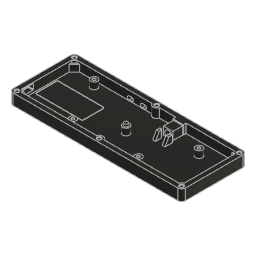
HTangl V2 Case (Autodesk Fusion 360 design; units mm, degrees)
Autodesk Fusion 360 part; units mm, degrees
sketch "Main Case" plane through (0, 0, 0) normal (0, 0, 1) x (1, 0, 0)
  line L0 (411.2, 144.2) -> (411.2, 21.8)
  line L1 (52.8, 13.8) -> (403.2, 13.8)
  line L2 (44.8, 21.8) -> (44.8, 144.2)
  circle A0 centre (228, 144.2) radius 3.3
  line L3 (237, 135.2) -> (219, 135.2)
  line L4 (237, 135.2) -> (237, 141)
  line L5 (219, 135.2) -> (219, 141)
  line L6 (403.2, 152.2) -> (52.8, 152.2)
  circle A1 centre (403.2, 144.2) radius 3.3
  line L7 (235.6916, 142) -> (395.5084, 142)
  arc A2 (395.5084, 142) -> (401, 136.5084) centre (403.2, 144.2) ccw
  arc A3 (411.2, 144.2) -> (403.2, 152.2) centre (403.2, 144.2) ccw
  arc A4 (220.3084, 142) -> (235.6916, 142) centre (228, 144.2) ccw
  circle A5 centre (52.8, 144.2) radius 3.3
  line L8 (220.3084, 142) -> (60.4916, 142)
  arc A6 (52.8, 152.2) -> (44.8, 144.2) centre (52.8, 144.2) ccw
  arc A7 (55, 136.5084) -> (60.4916, 142) centre (52.8, 144.2) ccw
  circle A8 centre (52.8, 21.8) radius 3.3
  line L9 (55, 136.5084) -> (55, 29.4916)
  arc A9 (44.8, 21.8) -> (52.8, 13.8) centre (52.8, 21.8) ccw
  arc A10 (60.4916, 24) -> (55, 29.4916) centre (52.8, 21.8) ccw
  circle A11 centre (403.2, 21.8) radius 3.3
  line L10 (401, 136.5084) -> (401, 29.4916)
  arc A12 (401, 29.4916) -> (395.5084, 24) centre (403.2, 21.8) ccw
  arc A13 (403.2, 13.8) -> (411.2, 21.8) centre (403.2, 21.8) ccw
  circle A14 centre (228, 21.8) radius 3.3
  line L11 (60.4916, 24) -> (220.3084, 24)
  line L12 (395.5084, 24) -> (235.6916, 24)
  arc A15 (235.6916, 24) -> (220.3084, 24) centre (228, 21.8) ccw
  line L13 (237, 30.8) -> (219, 30.8)
  line L14 (237, 30.8) -> (237, 25)
  line L15 (219, 30.8) -> (219, 25)
  line L16 (237, 141) -> (393, 141)
  line L17 (393, 141) -> (400, 134)
  line L18 (237, 25) -> (393, 25)
  line L19 (393, 25) -> (400, 32)
  line L20 (400, 32) -> (400, 134)
  line L21 (219, 25) -> (63, 25)
  line L22 (219, 141) -> (63, 141)
  line L23 (63, 141) -> (56, 134)
  line L24 (56, 134) -> (56, 32)
  line L25 (56, 32) -> (63, 25)
  point P0 (403.2, 144.2)
  point P1 (52.8, 144.2)
  point P2 (52.8, 21.8)
  point P3 (403.2, 21.8)
  dimension "d151" = 6.6
  dimension "d158" = 6.6
  dimension "d162" = 8
  dimension "d168" = 6.6
  dimension "d169" = 16
  dimension "d172" = 6.6
  dimension "d173" = 16
  dimension "d176" = 6.6
  dimension "d177" = 16
  dimension "d179" = 6.6
  dimension "d180" = 16
  dimension "d183" = 18
  dimension "d187" = 156
  dimension "d188" = 156
  dimension "d189" = 156
  dimension "d190" = 156
  dimension "d191" = 102
  constraint vertical L0
  constraint perpendicular L0 L1
  constraint perpendicular L1 L2
  constraint perpendicular L3 L4
  constraint perpendicular L3 L5
  constraint perpendicular L2 L6
  constraint coincident P0 A1.centre
  constraint horizontal L7
  constraint tangent L6 A3
  constraint tangent L0 A3
  constraint concentric A0 A4
  constraint coincident P1 A5.centre
  constraint concentric A5 A6
  constraint parallel L6 L8
  constraint coincident A7.start A6
  constraint concentric A6 A7
  constraint coincident P2 A8.centre
  constraint concentric A8 A9
  constraint coincident A10.start A9
  constraint concentric A9 A10
  constraint coincident P3 A11.centre
  constraint perpendicular L7 L10
  constraint concentric A12 A13
  constraint concentric A14 A15
  constraint horizontal L11
  constraint parallel L11 L12
  constraint perpendicular L13 L15
  constraint perpendicular L4 L16
  constraint perpendicular L14 L18
  constraint perpendicular L18 L20
  constraint perpendicular L15 L21
  constraint perpendicular L5 L22
  constraint perpendicular L22 L24
  measures "d151" diameter of A0
  measures "d158" diameter of A1
  measures "d162" radius of A3
  measures "d168" diameter of A5
  measures "d169" diameter of A6
  measures "d172" diameter of A8
  measures "d173" diameter of A9
  measures "d176" diameter of A11
  measures "d177" diameter of A12
  measures "d179" diameter of A14
  measures "d180" diameter of A15
  measures "d183" distance of L13.start L13.end
  measures "d187" distance of L4.end L16.end
  measures "d188" distance of L14.end L18.end
  measures "d189" distance of L15.end L21.end
  measures "d190" distance of L5.end L22.end
  measures "d191" distance of L23.end L24.end
extrude "Case Bottom" add sketch "Main Case" along normal blind 4.2 contours L3 L4 L5 L13 L14 L15 L16 L17 L18 L19 L20 L21 L22 L23 L24 L25 | L7 A2 A4 L8 A7 L9 A10 L10 A12 L11 L12 A15 makes body 1
sketch "Standoffs" plane through (0, 0, 4.2) normal (0, 0, 1) x (-1, 0, 0)
  circle A0 centre (-228, -79) radius 7.2
  circle A1 centre (-109, -130) radius 7.3
  circle A2 centre (-159, -35) radius 7.3
  circle A3 centre (-298, -35) radius 7.3
  circle A4 centre (-347, -115) radius 7.3
  circle A5 centre (-228, -79) radius 4.05
  circle A6 centre (-109, -130) radius 2.6
  circle A7 centre (-159, -35) radius 2.6
  circle A8 centre (-298, -35) radius 2.6
  circle A9 centre (-347, -115) radius 2.6
  point P0 (-228, -79)
  point P1 (-347, -115)
  point P2 (-298, -35)
  point P3 (-159, -35)
  point P4 (-109, -130)
  dimension "d35" = 14.4
  dimension "d36" = 14.6
  dimension "d37" = 14.6
  dimension "d38" = 14.6
  dimension "d39" = 14.6
  dimension "d41" = 8.1
  dimension "d62" = 5.2
  dimension "d63" = 5.2
  dimension "d64" = 5.2
  dimension "d65" = 5.2
  constraint coincident P0 A0.centre
  constraint coincident P4 A1.centre
  constraint coincident P3 A2.centre
  constraint coincident P2 A3.centre
  constraint coincident P1 A4.centre
  constraint concentric A2 A7
  constraint concentric A4 A9
  measures "d35" diameter of A0
  measures "d36" diameter of A1
  measures "d37" diameter of A2
  measures "d38" diameter of A3
  measures "d39" diameter of A4
  measures "d41" diameter of A5
  measures "d62" diameter of A6
  measures "d63" diameter of A7
  measures "d64" diameter of A8
  measures "d65" diameter of A9
extrude "Case Standoffs" add sketch "Standoffs" along normal blind 14.1 bodies 1
extrude "Center Post" add sketch "Standoffs" along normal blind 19.2 contours A5 bodies 1
extrude "Case Walls" add sketch "Main Case" along normal blind 23.4 contours L0 L1 L2 L6 A3 A6 A9 A13 bodies 1
extrude "PCB Mounting Holes" add 4 faces at (346.3647, 114.1522, 4.2) (297.2192, 35.376, 4.2) (159.7161, 35.7466, 4.2) (109.2885, 130.6201, 4.2) along direction (0, 0, 1) blind 10.2 on bodies 1 bodies 1
fillet "PCB Mounting Hole Fillet" radius 0.6 4 edges at (349.4241, 114.0598, 18.3) (300.4241, 34.0598, 18.3) (161.4241, 34.0598, 18.3) (111.4241, 129.0598, 18.3) on bodies 1
extrude "Top Panel Mounting Holes 1" add sketch "Main Case" along normal blind 12.6 contours A0 | A1 | A5 | A8 | A11 | A14 bodies 1
sketch "Top Panel Bolt Inset" plane through (0, 0, 23.4) normal (0, 0, 1) x (-1, 0, 0)
  line L0 (-60.4916, -142) -> (-220.3084, -142)
  arc A0 (-220.3084, -142) -> (-235.6916, -142) centre (-228, -144.2) ccw
  line L1 (-235.6916, -142) -> (-395.5084, -142)
  arc A1 (-395.5084, -142) -> (-401, -136.5084) centre (-403.2, -144.2) ccw
  line L2 (-401, -136.5084) -> (-401, -29.4916)
  arc A2 (-401, -29.4916) -> (-395.5084, -24) centre (-403.2, -21.8) ccw
  line L3 (-395.5084, -24) -> (-235.6916, -24)
  arc A3 (-235.6916, -24) -> (-220.3084, -24) centre (-228, -21.8) ccw
  line L4 (-220.3084, -24) -> (-60.4916, -24)
  arc A4 (-60.4916, -24) -> (-55, -29.4916) centre (-52.8, -21.8) ccw
  line L5 (-55, -29.4916) -> (-55, -136.5084)
  arc A5 (-55, -136.5084) -> (-60.4916, -142) centre (-52.8, -144.2) ccw
  circle A6 centre (-52.8, -144.2) radius 3.3
  circle A7 centre (-228, -144.2) radius 3.3
  circle A8 centre (-228, -21.8) radius 3.3
  circle A9 centre (-403.2, -144.2) radius 3.3
  circle A10 centre (-52.8, -21.8) radius 3.3
  circle A11 centre (-403.2, -21.8) radius 3.3
  arc A12 (-44.8, -21.8) -> (-52.8, -13.8) centre (-52.8, -21.8) ccw
  line L6 (-52.8, -13.8) -> (-403.2, -13.8)
  arc A13 (-403.2, -13.8) -> (-411.2, -21.8) centre (-403.2, -21.8) ccw
  line L7 (-411.2, -21.8) -> (-411.2, -144.2)
  arc A14 (-411.2, -144.2) -> (-403.2, -152.2) centre (-403.2, -144.2) ccw
  line L8 (-403.2, -152.2) -> (-52.8, -152.2)
  arc A15 (-52.8, -152.2) -> (-44.8, -144.2) centre (-52.8, -144.2) ccw
  line L9 (-44.8, -144.2) -> (-44.8, -21.8)
  circle A16 centre (-52.8, -144.2) radius 4.5
  circle A17 centre (-228, -144.2) radius 4.5
  circle A18 centre (-403.2, -144.2) radius 4.5
  circle A19 centre (-403.2, -21.8) radius 4.5
  circle A20 centre (-228, -21.8) radius 4.5
  circle A21 centre (-52.8, -21.8) radius 4.5
  dimension "d196" = 9
  dimension "d197" = 9
  dimension "d198" = 9
  dimension "d199" = 9
  dimension "d200" = 9
  dimension "d201" = 9
  constraint concentric A5 A16
  constraint concentric A0 A17
  constraint concentric A1 A18
  constraint concentric A2 A19
  constraint concentric A3 A20
  constraint concentric A4 A21
  measures "d196" diameter of A16
  measures "d197" diameter of A17
  measures "d198" diameter of A18
  measures "d199" diameter of A19
  measures "d200" diameter of A20
  measures "d201" diameter of A21
extrude "Top Panel Bolt Inset (1)" cut sketch "Top Panel Bolt Inset" against normal blind 1.2 contours A16 | A17 | A18 | A19 | A20 | A21 bodies 1
sketch "GC Port" plane through (0, 142, 0) normal (0, -1, 0) x (1, 0, 0)
  line L0 (235.6916, 4.2) -> (395.5084, 4.2)
  line L1 (395.5084, 4.2) -> (395.5084, 23.4)
  line L2 (235.6916, 23.4) -> (235.6916, 4.2)
  line L3 (271.55, 21.1) -> (291.45, 21.1)
  line L4 (271.55, 21.1) -> (271.55, 4.2)
  line L5 (291.45, 21.1) -> (291.45, 4.2)
  line L6 (291.45, 4.2) -> (291.45, 3.2)
  line L7 (271.55, 4.2) -> (271.55, 3.2)
  line L8 (291.45, 4.2) -> (271.55, 4.2)
  circle A0 centre (281.5, 11.25) radius 7.25
  line L9 (291.45, 3.2) -> (271.55, 3.2)
  line L10 (276.6624, 5.85) -> (286.3376, 5.85)
  point P0 (281.5, 6.05)
  point P1 (281.5, 5.85)
  dimension "d290" = 1
  dimension "d394" = 14.5
  dimension "d396" = 0.2
  constraint horizontal L3
  constraint coincident L0 L4.end
  constraint perpendicular L0 L4
  constraint coincident L0 L5.end
  constraint perpendicular L0 L5
  constraint perpendicular L7 L9
  constraint coincident A0 L10.start
  constraint coincident A0 L10.end
  constraint horizontal L10
  measures "d290" distance of L5.end L6.end
  measures "d394" diameter of A0
  measures "d396" distance of P0 P1
extrude "GC Port Cutout" cut sketch "GC Port" against normal blind 10.2 bodies 1
extrude "GC Port Surround" add sketch "GC Port" along normal blind 27 separate body contours L0 L3 L4 L5 L8 A0 | L0 L6 L7 L8 A0 L9 | L0 L8 A0 L10 | L0 L8 A0 makes body 2
extrude "GC Port Inset" cut sketch "GC Port" along normal blind 2.1 bodies 1 2
sketch "GC Port 2" plane through (0, 142, 0) normal (0, -1, 0) x (1, 0, 0)
  line L0 (271.55, 4.2) -> (271.55, 21.1)
  line L1 (271.55, 21.1) -> (291.45, 21.1)
  line L2 (291.45, 21.1) -> (291.45, 4.2)
  line L3 (291.45, 4.2) -> (395.5084, 4.2)
  line L4 (395.5084, 4.2) -> (395.5084, 23.4)
  line L5 (395.5084, 23.4) -> (235.6916, 23.4)
  line L6 (235.6916, 23.4) -> (235.6916, 4.2)
  line L7 (271.55, 21.1) -> (271.55, 4.2)
  line L8 (271.55, 21.1) -> (291.45, 21.1)
  line L9 (291.45, 21.1) -> (291.45, 4.2)
  line L10 (291.45, 4.2) -> (292.65, 4.2)
  line L11 (271.55, 4.2) -> (270.35, 4.2)
  line L12 (270.35, 4.2) -> (270.35, 23.4)
  line L13 (270.35, 23.4) -> (292.65, 23.4)
  line L14 (292.65, 23.4) -> (292.65, 4.2)
  line L15 (235.6916, 4.2) -> (271.55, 4.2)
  dimension "d322" = 1.2
  dimension "d323" = 1.2
  dimension "d324" = 22.3
  constraint coincident L0.end L1.start
  constraint coincident L1.end L2.start
  constraint coincident L0.start L7.end
  constraint coincident L2.end L3.start
  constraint perpendicular L9 L10
  constraint perpendicular L7 L11
  constraint coincident L5 L12.end
  constraint perpendicular L5 L12
  constraint perpendicular L12 L13
  measures "d322" distance of L2.end L10.end
  measures "d323" distance of L0.start L11.end
  measures "d324" distance of L12.end L13.end
extrude "GC Port Surround 2" add sketch "GC Port 2" along normal blind 6 contours L0 L1 L2 L3 L5 L7 L8 L9 L10 L11 L12 L13 L14 L15 bodies 1 2
sketch "GC Port 3" plane through (0, 152.2, 0) normal (0, 1, 0) x (-1, 0, 0)
  line L0 (-291.45, 3.2) -> (-291.45, 21.1)
  line L1 (-291.45, 21.1) -> (-271.55, 21.1)
  line L2 (-271.55, 21.1) -> (-271.55, 3.2)
  line L3 (-403.2, 0) -> (-52.8, 0)
  line L4 (-52.8, 0) -> (-52.8, 23.4)
  line L5 (-52.8, 23.4) -> (-403.2, 23.4)
  line L6 (-403.2, 23.4) -> (-403.2, 0)
  line L7 (-288.45, 21.1) -> (-274.55, 21.1)
  line L8 (-271.55, 18.1) -> (-271.55, 4.2)
  line L9 (-272.55, 3.2) -> (-290.45, 3.2)
  line L10 (-291.45, 4.2) -> (-291.45, 18.1)
  arc A0 (-288.45, 21.1) -> (-291.45, 18.1) centre (-288.45, 18.1) ccw
  arc A1 (-271.55, 18.1) -> (-274.55, 21.1) centre (-274.55, 18.1) ccw
  arc A2 (-291.45, 4.2) -> (-290.45, 3.2) centre (-290.45, 4.2) ccw
  arc A3 (-272.55, 3.2) -> (-271.55, 4.2) centre (-272.55, 4.2) ccw
  line L11 (-271.55, 3.2) -> (-291.45, 3.2)
  dimension "d364" = 3
  dimension "d365" = 1
  constraint horizontal L7
  constraint vertical L8
  constraint horizontal L9
  constraint vertical L10
  constraint tangent L7 A0
  constraint tangent L10 A0
  constraint tangent L7 A1
  constraint tangent L8 A1
  constraint equal A0 A1
  constraint tangent L9 A2
  constraint tangent L10 A2
  constraint tangent L8 A3
  constraint tangent L9 A3
  constraint equal A2 A3
  measures "d364" radius of A0
  measures "d365" radius of A2
extrude "Round corners of GC port hole" add sketch "GC Port 3" against normal blind 12.3 contours L0 A2 L11 | L0 L1 A0 | L2 A3 L11 | L1 L2 A1 bodies 1
sketch "GC Port Stopper" plane through (0, 0, 4.2) normal (0, 0, 1) x (-1, 0, 0)
  circle A0 centre (-109, -130) radius 7.3
  circle A1 centre (-159, -35) radius 7.3
  line L0 (-220.3084, -142) -> (-60.4916, -142)
  arc A2 (-55, -136.5084) -> (-60.4916, -142) centre (-52.8, -144.2) ccw
  line L1 (-55, -136.5084) -> (-55, -29.4916)
  arc A3 (-60.4916, -24) -> (-55, -29.4916) centre (-52.8, -21.8) ccw
  line L2 (-60.4916, -24) -> (-220.3084, -24)
  arc A4 (-235.6916, -24) -> (-220.3084, -24) centre (-228, -21.8) ccw
  line L3 (-235.6916, -24) -> (-395.5084, -24)
  arc A5 (-401, -29.4916) -> (-395.5084, -24) centre (-403.2, -21.8) ccw
  line L4 (-401, -29.4916) -> (-401, -136.5084)
  arc A6 (-395.5084, -142) -> (-401, -136.5084) centre (-403.2, -144.2) ccw
  line L5 (-270.35, -142) -> (-235.6916, -142)
  arc A7 (-220.3084, -142) -> (-235.6916, -142) centre (-228, -144.2) ccw
  circle A8 centre (-228, -79) radius 7.2
  circle A9 centre (-298, -35) radius 7.3
  circle A10 centre (-347, -115) radius 7.3
  line L6 (-271.55, -111) -> (-291.45, -111)
  line L7 (-291.45, -111) -> (-291.45, -108)
  line L8 (-291.45, -108) -> (-271.55, -108)
  line L9 (-271.55, -108) -> (-271.55, -111)
  line L10 (-271.55, -108) -> (-271.35, -108)
  line L11 (-271.55, -108) -> (-271.55, -107.8)
  line L12 (-271.35, -111) -> (-268.35, -111)
  line L13 (-268.35, -111) -> (-268.35, -103.2)
  line L14 (-271.35, -111) -> (-271.35, -107.8)
  line L15 (-271.35, -107.8) -> (-274.25, -107.8)
  line L16 (-274.25, -107.8) -> (-274.25, -103.2)
  line L17 (-274.25, -103.2) -> (-268.35, -103.2)
  line L18 (-291.45, -108) -> (-291.65, -108)
  line L19 (-291.45, -108) -> (-291.45, -107.8)
  line L20 (-291.65, -111) -> (-294.65, -111)
  line L21 (-291.65, -111) -> (-291.65, -107.8)
  line L22 (-291.65, -107.8) -> (-288.75, -107.8)
  line L23 (-288.75, -107.8) -> (-288.75, -103.2)
  line L24 (-288.75, -103.2) -> (-294.65, -103.2)
  line L25 (-294.65, -103.2) -> (-294.65, -111)
  line L26 (-270.35, -136) -> (-270.35, -142)
  line L27 (-395.5084, -142) -> (-292.65, -142)
  line L28 (-292.65, -142) -> (-292.65, -136)
  line L29 (-292.65, -136) -> (-291.45, -136)
  line L30 (-291.45, -136) -> (-291.45, -115)
  line L31 (-291.45, -115) -> (-271.55, -115)
  line L32 (-271.55, -115) -> (-271.55, -136)
  line L33 (-271.55, -136) -> (-270.35, -136)
  point P0 (-271.55, -115)
  point P1 (-291.45, -115)
  point P2 (-288.75, -108)
  point P3 (-274.25, -108)
  dimension "d303" = 4
  dimension "d305" = 3
  dimension "d306" = 0.2
  dimension "d307" = 0.2
  dimension "d308" = 3
  dimension "d309" = 7.8
  dimension "d312" = 0.2
  dimension "d313" = 0.2
  dimension "d314" = 3
  constraint horizontal L6
  constraint vertical L7
  constraint horizontal L8
  constraint vertical L9
  constraint perpendicular L9 L10
  constraint perpendicular L8 L11
  constraint perpendicular L12 L13
  constraint perpendicular L14 L15
  constraint perpendicular L15 L16
  constraint perpendicular L13 L17
  constraint perpendicular L7 L18
  constraint perpendicular L8 L19
  constraint perpendicular L7 L20
  constraint perpendicular L20 L21
  constraint perpendicular L21 L22
  constraint perpendicular L17 L23
  constraint perpendicular L23 L24
  constraint perpendicular L20 L25
  measures "d303" distance of P0 L6.start
  measures "d305" distance of L6.start L8.end
  measures "d306" distance of L8.end L10.end
  measures "d307" distance of L8.end L11.end
  measures "d308" distance of L12.start L12.end
  measures "d309" distance of L12.end L13.end
  measures "d312" distance of L7.end L18.end
  measures "d313" distance of L7.end L19.end
  measures "d314" distance of L20.start L20.end
extrude "GC Port Stopper (1)" add sketch "GC Port Stopper" along normal blind 14.1 contours L12 L13 L14 L15 L16 L17 | L20 L21 L22 L23 L24 L25 bodies 1
sketch "GC Port Stopper R" plane through (294.65, 0, 0) normal (1, 0, 0) x (0, 1, 0)
  line L0 (103.2, 4.2) -> (111, 4.2)
  line L1 (111, 4.2) -> (111, 18.3)
  line L2 (111, 18.3) -> (103.2, 18.3)
  line L3 (103.2, 18.3) -> (103.2, 4.2)
  line L4 (103.2, 18.3) -> (95.0594, 4.2)
  line L5 (103.2, 18.3) -> (119.4813, 18.3) construction
  line L6 (95.0594, 4.2) -> (103.2, 4.2)
  line L7 (103.2, 18.3) -> (103.2, 4.2)
  dimension "d317" = 120
  constraint horizontal L5
  constraint coincident L2.end L3.start
  constraint coincident L0.start L3.end
  constraint perpendicular L3 L6
  measures "d317" angle of L4 L5
extrude "GC Port Stopper R (1)" add sketch "GC Port Stopper R" against normal blind 5.9 separate body contours L3 L4 L6 L7 makes body 3
sketch "GC Port Stopper L" plane through (268.35, 0, 0) normal (-1, 0, 0) x (0, -1, 0)
  line L0 (-111, 4.2) -> (-103.2, 4.2)
  line L1 (-103.2, 4.2) -> (-103.2, 18.3)
  line L2 (-103.2, 18.3) -> (-111, 18.3)
  line L3 (-111, 18.3) -> (-111, 4.2)
  line L4 (-103.2, 18.3) -> (-103.2, 4.2)
  line L5 (-103.2, 18.3) -> (-95.0594, 4.2)
  line L6 (-95.0594, 4.2) -> (-103.2, 4.2)
  dimension "d329" = 150
  constraint coincident L1.end L2.start
  constraint coincident L0.end L1.start
  constraint perpendicular L1 L6
  measures "d329" angle of L4 L5
extrude "GC Port Stopper L (1)" add sketch "GC Port Stopper L" against normal blind 5.9 separate body contours L1 L4 L5 L6 makes body 4
combine "Join GC Port Supports To Case" operation add target body 4 tool bodies 3 1
sketch "USB Ports" plane through (0, 152.2, 0) normal (0, 1, 0) x (-1, 0, 0)
  line L0 (-272.55, 3.2) -> (-290.45, 3.2)
  line L1 (-291.45, 4.2) -> (-291.45, 18.1)
  line L2 (-288.45, 21.1) -> (-274.55, 21.1)
  line L3 (-271.55, 18.1) -> (-271.55, 4.2)
  line L4 (-403.2, 0) -> (-52.8, 0)
  line L5 (-52.8, 0) -> (-52.8, 23.4)
  line L6 (-52.8, 23.4) -> (-403.2, 23.4)
  line L7 (-403.2, 23.4) -> (-403.2, 0)
  line L8 (-204.5, 13.05) -> (-199.5, 13.05)
  line L9 (-195.5, 9.05) -> (-195.5, 9.05)
  line L10 (-199.5, 5.05) -> (-204.5, 5.05)
  line L11 (-208.5, 9.05) -> (-208.5, 9.05)
  arc A0 (-204.5, 13.05) -> (-208.5, 9.05) centre (-204.5, 9.05) ccw
  arc A1 (-199.5, 5.05) -> (-195.5, 9.05) centre (-199.5, 9.05) ccw
  arc A2 (-195.5, 9.05) -> (-199.5, 13.05) centre (-199.5, 9.05) ccw
  arc A3 (-208.5, 9.05) -> (-204.5, 5.05) centre (-204.5, 9.05) ccw
  line L12 (-176.5, 13.05) -> (-171.5, 13.05)
  line L13 (-167.5, 9.05) -> (-167.5, 9.05)
  line L14 (-171.5, 5.05) -> (-176.5, 5.05)
  line L15 (-180.5, 9.05) -> (-180.5, 9.05)
  arc A4 (-176.5, 13.05) -> (-180.5, 9.05) centre (-176.5, 9.05) ccw
  arc A5 (-167.5, 9.05) -> (-171.5, 13.05) centre (-171.5, 9.05) ccw
  arc A6 (-180.5, 9.05) -> (-176.5, 5.05) centre (-176.5, 9.05) ccw
  arc A7 (-171.5, 5.05) -> (-167.5, 9.05) centre (-171.5, 9.05) ccw
  arc A8 (-291.45, 4.2) -> (-290.45, 3.2) centre (-290.45, 4.2) ccw
  arc A9 (-288.45, 21.1) -> (-291.45, 18.1) centre (-288.45, 18.1) ccw
  arc A10 (-271.55, 18.1) -> (-274.55, 21.1) centre (-274.55, 18.1) ccw
  arc A11 (-272.55, 3.2) -> (-271.55, 4.2) centre (-272.55, 4.2) ccw
  arc A12 (-291.45, 4.2) -> (-290.45, 3.2) centre (-290.45, 4.2) ccw
  line L16 (-291.45, 4.2) -> (-291.45, 18.1)
  arc A13 (-288.45, 21.1) -> (-291.45, 18.1) centre (-288.45, 18.1) ccw
  line L17 (-288.45, 21.1) -> (-274.55, 21.1)
  arc A14 (-271.55, 18.1) -> (-274.55, 21.1) centre (-274.55, 18.1) ccw
  line L18 (-271.55, 18.1) -> (-271.55, 4.2)
  arc A15 (-272.55, 3.2) -> (-271.55, 4.2) centre (-272.55, 4.2) ccw
  line L19 (-403.2, 0) -> (-52.8, 0)
  line L20 (-52.8, 0) -> (-52.8, 23.4)
  line L21 (-52.8, 23.4) -> (-403.2, 23.4)
  line L22 (-403.2, 23.4) -> (-403.2, 0)
  line L23 (-272.55, 3.2) -> (-290.45, 3.2)
  point P0 (-202, 23.4)
  point P1 (-174, 23.4)
  point P2 (-228, 23.4)
  point P3 (-281.5, 21.1)
  point P4 (-202, 9.05)
  point P5 (-174, 9.05)
  point P6 (-202, 9.05)
  point P7 (-174, 9.05)
  point P8 (-208.5, 13.05)
  point P9 (-195.5, 13.05)
  point P10 (-195.5, 5.05)
  point P11 (-208.5, 5.05)
  point P12 (-180.5, 13.05)
  point P13 (-167.5, 13.05)
  point P14 (-167.5, 5.05)
  point P15 (-180.5, 5.05)
  dimension "d334" = 14.35
  dimension "d335" = 14.35
  dimension "d336" = 13
  dimension "d337" = 8
  dimension "d338" = 13
  dimension "d339" = 8
  dimension "d340" = 4
  dimension "d341" = 4
  dimension "d342" = 4
  dimension "d343" = 4
  dimension "d344" = 4
  dimension "d345" = 4
  dimension "d346" = 4
  dimension "d347" = 4
  constraint midpoint L6 P2
  constraint midpoint L2 P3
  constraint coincident P6 P4
  constraint coincident P7 P5
  constraint horizontal L8
  constraint tangent L8 A0
  constraint tangent L10 A1
  constraint tangent L8 A2
  constraint tangent L10 A3
  constraint horizontal L12
  constraint tangent L12 A4
  constraint tangent L12 A5
  constraint tangent L14 A6
  constraint tangent L14 A7
  measures "d334" distance of P0 P6
  measures "d335" distance of P1 P7
  measures "d336" distance of P10 P11
  measures "d337" distance of P8 P11
  measures "d338" distance of P12 P13
  measures "d339" distance of P12 P15
  measures "d340" radius of A0
  measures "d341" radius of A1
  measures "d342" radius of A2
  measures "d343" radius of A3
  measures "d344" radius of A4
  measures "d345" radius of A5
  measures "d346" radius of A6
  measures "d347" radius of A7
extrude "USB Ports (1)" cut sketch "USB Ports" against normal blind 10.2 contours L8 L10 A0 A1 A2 A3 | L12 L14 A4 A5 A6 A7 bodies 4
sketch "Nunchuk Port" plane through (44.8, 0, 0) normal (-1, 0, 0) x (0, -1, 0)
  line L0 (-55, 20.3) -> (-55, 10.3)
  line L1 (-33, 20.3) -> (-33, 10.3)
  line L2 (-54, 21.3) -> (-34, 21.3)
  line L3 (-54, 9.3) -> (-34, 9.3)
  arc A0 (-54, 21.3) -> (-55, 20.3) centre (-54, 20.3) ccw
  arc A1 (-33, 20.3) -> (-34, 21.3) centre (-34, 20.3) ccw
  arc A2 (-34, 9.3) -> (-33, 10.3) centre (-34, 10.3) ccw
  arc A3 (-55, 10.3) -> (-54, 9.3) centre (-54, 10.3) ccw
  dimension "d420" = 1
  constraint perpendicular L1 L2
  constraint perpendicular L1 L3
  constraint tangent L2 A0
  constraint tangent L0 A0
  constraint tangent L2 A1
  constraint tangent L1 A1
  constraint equal A0 A1
  constraint tangent L1 A2
  constraint tangent L3 A2
  constraint equal A0 A2
  constraint tangent L0 A3
  constraint tangent L3 A3
  constraint equal A0 A3
  measures "d420" radius of A0
extrude "Nunchuk Hole" cut sketch "Nunchuk Port" against normal blind 10.2 bodies 4
sketch "Brook Board Inset" plane through (0, 0, 4.2) normal (0, 0, 1) x (-1, 0, 0)
  circle A0 centre (-109, -130) radius 7.3
  circle A1 centre (-159, -35) radius 7.3
  circle A2 centre (-228, -79) radius 7.2
  circle A3 centre (-298, -35) radius 7.3
  circle A4 centre (-347, -115) radius 7.3
  line L0 (-270.35, -136) -> (-270.35, -142)
  line L1 (-270.35, -142) -> (-235.6916, -142)
  arc A5 (-220.3084, -142) -> (-235.6916, -142) centre (-228, -144.2) ccw
  line L2 (-220.3084, -142) -> (-60.4916, -142)
  arc A6 (-55, -136.5084) -> (-60.4916, -142) centre (-52.8, -144.2) ccw
  line L3 (-55, -136.5084) -> (-55, -29.4916)
  arc A7 (-60.4916, -24) -> (-55, -29.4916) centre (-52.8, -21.8) ccw
  line L4 (-60.4916, -24) -> (-220.3084, -24)
  arc A8 (-235.6916, -24) -> (-220.3084, -24) centre (-228, -21.8) ccw
  line L5 (-235.6916, -24) -> (-395.5084, -24)
  arc A9 (-401, -29.4916) -> (-395.5084, -24) centre (-403.2, -21.8) ccw
  line L6 (-401, -29.4916) -> (-401, -136.5084)
  arc A10 (-395.5084, -142) -> (-401, -136.5084) centre (-403.2, -144.2) ccw
  line L7 (-395.5084, -142) -> (-292.65, -142)
  line L8 (-292.65, -142) -> (-292.65, -136)
  line L9 (-292.65, -136) -> (-291.45, -136)
  line L10 (-291.45, -136) -> (-291.45, -115)
  line L11 (-291.45, -115) -> (-271.55, -115)
  line L12 (-271.55, -115) -> (-271.55, -136)
  line L13 (-271.55, -136) -> (-270.35, -136)
  line L14 (-274.25, -107.8) -> (-274.25, -95.0594)
  line L15 (-274.25, -95.0594) -> (-268.35, -95.0594)
  line L16 (-268.35, -95.0594) -> (-268.35, -111)
  line L17 (-268.35, -111) -> (-271.35, -111)
  line L18 (-271.35, -111) -> (-271.35, -107.8)
  line L19 (-271.35, -107.8) -> (-274.25, -107.8)
  line L20 (-288.75, -95.0594) -> (-288.75, -107.8)
  line L21 (-288.75, -107.8) -> (-291.65, -107.8)
  line L22 (-291.65, -107.8) -> (-291.65, -111)
  line L23 (-291.65, -111) -> (-294.65, -111)
  line L24 (-294.65, -111) -> (-294.65, -95.0594)
  line L25 (-294.65, -95.0594) -> (-288.75, -95.0594)
  line L26 (-60, -103) -> (-156, -103)
  line L27 (-158, -101) -> (-158, -58)
  line L28 (-156, -56) -> (-60, -56)
  line L29 (-58, -58) -> (-58, -101)
  arc A11 (-158, -101) -> (-156, -103) centre (-156, -101) ccw
  arc A12 (-60, -103) -> (-58, -101) centre (-60, -101) ccw
  arc A13 (-58, -58) -> (-60, -56) centre (-60, -58) ccw
  arc A14 (-156, -56) -> (-158, -58) centre (-156, -58) ccw
  dimension "d368" = 2
  constraint horizontal L26
  constraint vertical L27
  constraint horizontal L28
  constraint vertical L29
  constraint tangent L26 A11
  constraint tangent L27 A11
  constraint tangent L26 A12
  constraint tangent L29 A12
  constraint equal A11 A12
  constraint tangent L28 A13
  constraint tangent L29 A13
  constraint equal A11 A13
  constraint tangent L27 A14
  constraint tangent L28 A14
  constraint equal A11 A14
  measures "d368" radius of A11
extrude "Brook Board Inset (1)" cut sketch "Brook Board Inset" against normal blind 0.6 contours L26 L27 L28 L29 A11 A12 A13 A14 bodies 4
sketch "PCB Supports" plane through (0, 0, 4.2) normal (0, 0, 1) x (-1, 0, 0)
  line L0 (-156, -56) -> (-60, -56)
  arc A0 (-58, -58) -> (-60, -56) centre (-60, -58) ccw
  line L1 (-58, -58) -> (-58, -101)
  arc A1 (-60, -103) -> (-58, -101) centre (-60, -101) ccw
  line L2 (-60, -103) -> (-156, -103)
  arc A2 (-158, -101) -> (-156, -103) centre (-156, -101) ccw
  line L3 (-158, -101) -> (-158, -58)
  arc A3 (-156, -56) -> (-158, -58) centre (-156, -58) ccw
  circle A4 centre (-109, -130) radius 7.3
  circle A5 centre (-159, -35) radius 7.3
  circle A6 centre (-228, -79) radius 7.2
  circle A7 centre (-298, -35) radius 7.3
  circle A8 centre (-347, -115) radius 7.3
  line L4 (-270.35, -136) -> (-270.35, -142)
  line L5 (-270.35, -142) -> (-235.6916, -142)
  arc A9 (-220.3084, -142) -> (-235.6916, -142) centre (-228, -144.2) ccw
  line L6 (-220.3084, -142) -> (-60.4916, -142)
  arc A10 (-55, -136.5084) -> (-60.4916, -142) centre (-52.8, -144.2) ccw
  line L7 (-55, -136.5084) -> (-55, -29.4916)
  arc A11 (-60.4916, -24) -> (-55, -29.4916) centre (-52.8, -21.8) ccw
  line L8 (-60.4916, -24) -> (-220.3084, -24)
  arc A12 (-235.6916, -24) -> (-220.3084, -24) centre (-228, -21.8) ccw
  line L9 (-235.6916, -24) -> (-395.5084, -24)
  arc A13 (-401, -29.4916) -> (-395.5084, -24) centre (-403.2, -21.8) ccw
  line L10 (-401, -29.4916) -> (-401, -136.5084)
  arc A14 (-395.5084, -142) -> (-401, -136.5084) centre (-403.2, -144.2) ccw
  line L11 (-395.5084, -142) -> (-292.65, -142)
  line L12 (-292.65, -142) -> (-292.65, -136)
  line L13 (-292.65, -136) -> (-291.45, -136)
  line L14 (-291.45, -136) -> (-291.45, -115)
  line L15 (-291.45, -115) -> (-271.55, -115)
  line L16 (-271.55, -115) -> (-271.55, -136)
  line L17 (-271.55, -136) -> (-270.35, -136)
  line L18 (-274.25, -107.8) -> (-274.25, -95.0594)
  line L19 (-274.25, -95.0594) -> (-268.35, -95.0594)
  line L20 (-268.35, -95.0594) -> (-268.35, -111)
  line L21 (-268.35, -111) -> (-271.35, -111)
  line L22 (-271.35, -111) -> (-271.35, -107.8)
  line L23 (-271.35, -107.8) -> (-274.25, -107.8)
  line L24 (-288.75, -95.0594) -> (-288.75, -107.8)
  line L25 (-288.75, -107.8) -> (-291.65, -107.8)
  line L26 (-291.65, -107.8) -> (-291.65, -111)
  line L27 (-291.65, -111) -> (-294.65, -111)
  line L28 (-294.65, -111) -> (-294.65, -95.0594)
  line L29 (-294.65, -95.0594) -> (-288.75, -95.0594)
  line L30 (-395.4218, -29.5782) -> (-401, -35.1563)
  line L31 (-395.4218, -29.5782) -> (-389.8437, -24)
  line L32 (-389.8434, -142) -> (-401, -130.8434)
  line L33 (-57.665, -32.4916) -> (-66.1566, -24)
  line L34 (-66.1566, -142) -> (-55, -130.8434)
  line L35 (-55, -32.4916) -> (-57.665, -32.4916)
  constraint coincident L10 L30.end
  constraint coincident L9 L31.end
  constraint perpendicular L7 L35
extrude "PCB Supports Extrude" add sketch "PCB Supports" along normal blind 14.1 contours L6 A10 L7 L34 | L7 A11 L8 L33 L35 | L10 A14 L11 L32 | L9 A13 L10 L30 L31 bodies 4
named bodies: "Case", "GC Bracket", "GC Port Support R"
